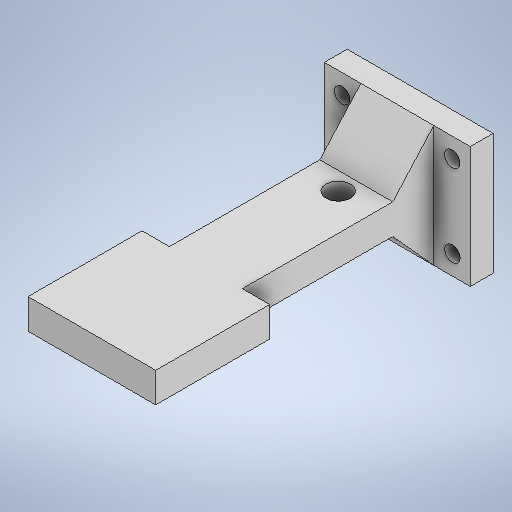
# Autodesk Inventor part: Actuator
Saved by Autodesk Inventor 2025.1 (Build 291241000, 241)
## iProperties
Created: 2025-01-26
Part Number: Actuator
Material: Generic
Document SubType Name: Modeling
Designer: 13156
Density: 1 g/cm^3
Appearance: Default
Author: 13156
Autodesk Inventor part; units mm, degrees
ref_plane "YZ Plane" through (0, 0, 0) normal (1, 0, 0) x (0, 1, 0)
ref_plane "XZ Plane" through (0, 0, 0) normal (0, 1, 0) x (-1, 0, 0)
ref_plane "XY Plane" through (0, 0, 0) normal (0, 0, 1) x (1, 0, 0)
sketch "Sketch1" plane through (0, 0, 0) normal (0, 0, 1) x (1, 0, 0)
  line L0 (-16, 5) -> (16, 5)
  line L1 (16, 5) -> (16, -5)
  line L2 (16, -5) -> (-16, -5)
  line L3 (-16, -5) -> (-16, 5)
  line L4 (0, 1.062) -> (0, -0.494) construction
  line L5 (-13.0353, 0) -> (11.6638, 0) construction
  line L6 (0, -7) -> (0, 7) projected
  line L7 (-22.4, 0) -> (22.4, 0) projected
  point P0 (0, 0)
  dimension "d0" = 32
  dimension "d1" = 10
  constraints: 12 end point, 2 horizontal, 2 parallel, 2 perpendicular, 2 other
  measures "d0" distance of L0.start L0.end
  measures "d1" distance of L0.end L1.end
extrude "Extrusion1" add sketch "Sketch1" along normal blind 5
sketch "Sketch2" plane through (0, 0, 5) normal (0, 0, 1) x (1, 0, 0)
  circle A0 centre (-12.1, -0.7125) radius 1.7
  circle A1 centre (12.1, -0.7125) radius 1.7
  line L0 (0, -7) -> (0, 7) projected
  line L1 (16, 5) -> (-16, 5) projected
  point P0 (0, 0)
  dimension "d4" = 3.4
  dimension "d5" = 24.2
  dimension "d38" = 5.7125
  constraints: 2 centre point, 1 equal radius, 1 symmetric about line
  measures "d4" diameter of A1
  measures "d5" distance of A0.centre A1.centre
  measures "d38" distance from line of L1 A1.centre
extrude "Extrusion2" cut sketch "Sketch2" against normal blind 6.575
sketch "Sketch3" plane through (-16, 5, 0) normal (0, 1, 0) x (1, 0, 0)
  line L0 (32, -5) -> (0, -5) projected
  line L1 (32, 0) -> (0, 0) projected
  line L2 (0, 0) -> (32, 0)
  line L3 (0, 0) -> (0, -10)
  line L4 (0, -10) -> (8, -10)
  line L5 (32, -10) -> (24, -10)
  line L6 (24, -10) -> (24, -47)
  line L7 (24, -47) -> (30, -47)
  line L8 (30, -47) -> (30, -72)
  line L9 (30, -72) -> (2, -72)
  line L10 (2, -72) -> (2, -47)
  line L11 (2, -47) -> (8, -47)
  line L12 (8, -47) -> (8, -10)
  line L13 (32, 0) -> (32, -5) projected
  line L14 (16, 7.4504) -> (16, -44.7023) projected
  line L15 (32, -10) -> (32, 0)
  point P0 (16, 0)
  dimension "d8" = 10
  dimension "d9" = 37
  dimension "d10" = 25
  dimension "d11" = 8
  dimension "d12" = 28
  constraints: 24 end point, 7 perpendicular, 2 point on line, 2 vertical, 1 collinear, 5 other
  measures "d8" distance of L1.end L3.end
  measures "d9" distance of L11.end L4.end
  measures "d10" distance of L9.end L10.end
  measures "d11" distance of L5.start L5.end
  measures "d12" distance of L8.end L9.end
extrude "Extrusion3" add sketch "Sketch3" along normal blind 6.575
sketch "Sketch4" plane through (-16, 5, 0) normal (0, -1, 0) x (1, 0, 0)
  circle A0 centre (16, 17.954) radius 2.7
  line L0 (0, 5) -> (32, 5) projected
  line L1 (24, 10) -> (32, 10) projected
  point P0 (16, 0)
  point P1 (16, 5)
  dimension "d15" = 12.954
  dimension "d16" = 5.4
  dimension "d17" = 7.954
  constraints: 1 centre point, 1 midpoint
  measures "d15" distance of point (16, 5) A0.centre
  measures "d16" diameter of A0
  measures "d17" distance from line of L1 A0.centre
extrude "Extrusion4" cut sketch "Sketch4" against normal blind 6.575
sketch "Sketch5" plane through (0, 0, 5) normal (0, 0, 1) x (1, 0, 0)
  line L0 (-16, -5) -> (-16, 11.575) projected
  line L1 (-16, 11.575) -> (16, 11.575)
  line L2 (16, 11.575) -> (16, 21.575)
  line L3 (16, 21.575) -> (-16, 21.575)
  line L4 (-16, 21.575) -> (-16, 11.575)
  line L5 (16, -5) -> (16, 5) projected
  point P0 (0, 0)
  point P1 (-16, 16.575)
  dimension "d23" = 32
  constraints: 8 end point, 2 parallel, 1 collinear, 1 horizontal, 1 midpoint, 1 perpendicular
  measures "d23" distance from line of point (-16, 16.575) L2
extrude "Extrusion5" add sketch "Sketch5" against normal up to surface (5 mm away)
sketch "Sketch6" plane through (0, 0, 0) normal (0, 0, -1) x (-1, 0, 0)
  circle A0 centre (-12.0486, 17.2875) radius 1.7
  circle A1 centre (12.1, 17.2875) radius 1.7
  circle A2 centre (-12.1, -0.7125) radius 1.7 projected
  circle A3 centre (12.1, -0.7125) radius 1.7 projected
  point P0 (0, 0)
  dimension "d26" = 18
  dimension "d27" = 0
  dimension "d28" = 0
  dimension "d29" = 0.0514
  constraints: 2 centre point, 2 equal radius
  measures "d26" vertical distance of A2.centre A0.centre
  measures "d27" vertical distance of A0.centre A1.centre
  measures "d28" horizontal distance of A3.centre A1.centre
  measures "d29" horizontal distance of A2.centre A0.centre
extrude "Extrusion6" cut sketch "Sketch6" against normal blind 10 contours A0 | A1
sketch "Sketch7" plane through (-16, 11.575, 0) normal (0, 1, 0) x (1, 0, 0)
  line L0 (32, -5) -> (0, -5) projected
  line L1 (8, -10) -> (8, -47) projected
  line L2 (24, -5) -> (8, -5)
  line L3 (8, -5) -> (8, -14)
  line L4 (8, -14) -> (24, -14)
  line L5 (24, -14) -> (24, -5)
  line L6 (24, -47) -> (24, -10) projected
  point P0 (16, 0)
  dimension "d39" = 0
  dimension "d40" = 9
  constraints: 8 end point, 2 parallel, 2 point on line, 1 horizontal, 1 perpendicular
  measures "d39" distance between parallel lines of L6 L5
  measures "d40" distance between parallel lines of L0 L4
extrude "Extrusion7" add sketch "Sketch7" along normal blind 10 and the other way blind 16.575
chamfer "Chamfer4" distance 9 distance2 10 1 edges at (0, 21.575, 14) measured on face at (0, 21.575, 13.5)
chamfer "Chamfer5" distance 9 distance2 10 1 edges at (0, -5, 14) measured on face at (0, -5, 13.5)
sketch "Sketch8" plane through (-16, 11.575, 0) normal (0, 1, 0) x (1, 0, 0)
  line L0 (8, -10) -> (8, -5) projected
  line L1 (0, -5) -> (0, -10) projected
  line L2 (8, -5) -> (0, -5)
  line L3 (0, -5) -> (0, -10)
  line L4 (0, -10) -> (8, -10)
  line L5 (8, -10) -> (8, -5)
  line L6 (24, -5) -> (32, -5)
  line L7 (32, -5) -> (32, -10)
  line L8 (32, -10) -> (24, -10)
  line L9 (24, -10) -> (24, -5)
  line L10 (32, -10) -> (32, -5) projected
  line L11 (24, -14) -> (24, -5) projected
  point P0 (16, 0)
  dimension "d51" = 0
  dimension "d52" = 0
  constraints: 16 end point, 4 parallel, 2 horizontal, 2 perpendicular, 2 point on line
  measures "d51" distance between parallel lines of L10 L7
  measures "d52" distance between parallel lines of L11 L9
extrude "Extrusion8" cut sketch "Sketch8" against normal blind 10
body "Solid1"
